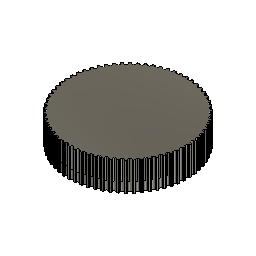
gear_66Z (Autodesk Fusion 360 design; units mm, degrees)
Autodesk Fusion 360 part; units mm, degrees
sketch "Sketch1" plane through (0, 0, 0) normal (0, 0, 1) x (1, 0, 0) in component "gt2 pulley"
  circle A0 centre (0, 0) radius 21.0085 construction
  circle A1 centre (0, 0) radius 20.0045 construction
  line L0 (0, 0) -> (0, 21.0085) construction
  line L1 (0, 0) -> (0.9996, 20.9847) construction
  line L2 (0, 0) -> (1.4058, 20.9614) construction
  circle A2 centre (0, 0) radius 20.7545 construction
  arc A3 (0.3929, 20.6167) -> (0.4663, 20.3219) centre (1.3888, 20.7079) ccw
  circle A4 centre (0, 0) radius 20.6045 construction
  arc A5 (0.2453, 20.753) -> (0, 20.7545) centre (0, 0) ccw
  arc A6 (0.3929, 20.6167) -> (0.2453, 20.753) centre (0.2436, 20.603) ccw
  arc A7 (0.4663, 20.3219) -> (0.9519, 19.9818) centre (0.9783, 20.5362) ccw
  arc A8 (0, 20.7545) -> (-0.2453, 20.753) centre (0, 0) ccw
  arc A9 (-0.2453, 20.753) -> (-0.3929, 20.6167) centre (-0.2436, 20.603) ccw
  arc A10 (-0.4663, 20.3219) -> (-0.3929, 20.6167) centre (-1.3888, 20.7079) ccw
  arc A11 (-0.9519, 19.9818) -> (-0.4663, 20.3219) centre (-0.9783, 20.5362) ccw
  arc A12 (0.9519, 19.9818) -> (-0.9519, 19.9818) centre (0, 0) ccw
  point P0 (1.3888, 20.7079)
  point P1 (0, 20.7545)
  dimension "d18" = 42.0169
  dimension "d19" = 2.727
  dimension "d22" = 1.004
  dimension "d24" = 0.75
  dimension "d26" = 1
  dimension "d27" = 0.15
  dimension "d28" = 0.15
  dimension "d47" = 0.555
  dimension "d52" = 3.812
  constraint coincident A0.centre A1.centre
  constraint coincident A0 L0.end
  constraint vertical L0
  constraint coincident A0 L1.end
  constraint coincident A0 L2.end
  constraint concentric A1 A2
  constraint coincident A1 A7.end
  constraint coincident L1 A7.end
  constraint coincident A2 P0
  constraint coincident L2 P0
  constraint coincident P0 A3.centre
  constraint coincident A2 P1
  constraint coincident L0 P1
  constraint concentric A2 A4
  constraint coincident P1 A5.end
  constraint coincident A4 A6.centre
  constraint coincident A3.start A6.start
  constraint tangent A3 A6
  constraint tangent A3 A7
  constraint symmetric L0 A7.end A11.start
  constraint symmetric L0 A3.start A9.end
  constraint symmetric L0 A3.end A10.start
  constraint symmetric L0 A3 A10
  constraint symmetric L0 A5.start A8.end
  constraint symmetric L0 P1 A5.end
  constraint symmetric L0 A5 A8
  constraint symmetric L0 A6 A9
  constraint symmetric L0 A7 A11
  constraint coincident A1 A11.start
  constraint tangent A1 A7
  constraint coincident L1 A7.centre
  measures "d18" diameter of A0
  measures "d19" angle of L0 L1
  measures "d22" distance of A0 A1
  measures "d24" distance of A1 A2
  measures "d26" radius of A3
  measures "d27" distance of A2 A4
  measures "d28" radius of A6
  measures "d47" radius of A7
extrude "Extrude4" [suppressed] in component "gt2 pulley"
pattern_circular "C-Pattern7" [suppressed] in component "gt2 pulley"
extrude "Extrude3" [suppressed] in component "gt2 pulley"
pattern_circular "C-Pattern6" [suppressed] in component "gt2 pulley"
extrude "Extrude2" [suppressed] in component "gt2 pulley"
pattern_circular "C-Pattern5" [suppressed] in component "gt2 pulley"
extrude "Extrude1" [suppressed] in component "gt2 pulley"
pattern_circular "C-Pattern4" [suppressed] in component "gt2 pulley"
pattern_circular "C-Pattern3" [suppressed] in component "gt2 pulley"
pattern_circular "C-Pattern2" [suppressed] in component "gt2 pulley"
pattern_circular "C-Pattern1" [suppressed] in component "gt2 pulley"
copy_body "Body->Comp1" [suppressed] in component "Component"
copy_body "Body->Comp2" [suppressed] in component "Component'"
copy_body "Body->Comp3" [suppressed] in component "Component''"
copy_body "Body->Comp4" [suppressed] in component "Component'''"
copy_body "Body->Comp5" [suppressed] in component "Component''''"
copy_body "Body->Comp6" [suppressed] in component "Component'''''"
copy_body "Body->Comp7" [suppressed] in component "Component''''''"
copy_body "Body->Comp8" [suppressed] in component "Component'''''''"
copy_body "Body->Comp9" [suppressed] in component "Component''''''''"
copy_body "Body->Comp10" [suppressed] in component "Component'''''''''"
copy_body "Body->Comp11" [suppressed] in component "Component''''''''''"
copy_body "Body->Comp12" [suppressed] in component "Component'''''''''''"
copy_body "Body->Comp13" [suppressed] in component "Component''''''''''''"
copy_body "Body->Comp14" [suppressed] in component "Component'''''''''''''"
copy_body "Body->Comp15" [suppressed] in component "Component''''''''''''''"
copy_body "Body->Comp16" [suppressed] in component "Component'''''''''''''''"
copy_body "Body->Comp17" [suppressed] in component "Component''''''''''''''''"
copy_body "Body->Comp18" [suppressed] in component "Component'''''''''''''''''"
copy_body "Body->Comp19" [suppressed] in component "Component''''''''''''''''''"
copy_body "Body->Comp20" [suppressed] in component "Component'''''''''''''''''''"
extrude "Extrude1'" add sketch "Sketch1" along normal blind 7 makes body 1
pattern_circular "C-Pattern1'" count 66 over 360 about axis through (0, 0, 1.75) along (0, 0, 1) of bodies 1 makes body 2 at (-2.0069, 19.9035, 4.6667) makes body 3 at (-3.8897, 19.6226, 4.6667) makes body 4 at (-5.7374, 19.164, 4.6667) makes body 5 at (-6.7424, 18.834, 2.3333) makes body 6 at (-9.2605, 17.7319, 4.6667) makes body 7 at (-10.1849, 17.2176, 2.3333) makes body 8 at (-11.7754, 16.1715, 2.3333) makes body 9 at (-13.2593, 14.9789, 2.3333) makes body 10 at (-14.6231, 13.6507, 2.3333) makes body 11 at (-15.8545, 12.1989, 2.3333) makes body 12 at (-17.377, 9.9104, 4.6667) makes body 13 at (-18.2404, 8.2138, 4.6667) makes body 14 at (-19.1335, 5.8386, 4.6667) makes body 15 at (-19.4652, 4.6133, 4.6667) makes body 16 at (-19.6819, 3.5779, 2.3333) makes body 17 at (-19.9866, 0.8461, 4.6667) makes body 18 at (-19.9765, -1.0576, 4.6667) makes body 19 at (-19.7855, -2.9517, 4.6667) makes body 20 at (-19.2527, -5.4326, 4.6667) makes body 21 at (-19.1334, -5.8386, 2.3333) makes body 22 at (-17.8766, -8.978, 4.6667) makes body 23 at (-16.9422, -10.6367, 4.6667) makes body 24 at (-16.7135, -10.9926, 2.3333) makes body 25 at (-14.6231, -13.6508, 4.6667) makes body 26 at (-13.7279, -14.5507, 4.6667) makes body 27 at (-11.7754, -16.1715, 4.6667) makes body 28 at (-10.1849, -17.2176, 4.6667) makes body 29 at (-9.0724, -17.8289, 4.6667) makes body 30 at (-6.7424, -18.834, 4.6667) makes body 31 at (-5.5343, -19.2237, 4.6667) makes body 32 at (-4.5103, -19.4894, 2.3333) makes body 33 at (-1.7962, -19.9237, 4.6667) makes body 34 at (0.1058, -20.0042, 4.6667) makes body 35 at (2.6374, -19.8298, 4.6667) makes body 36 at (3.8897, -19.6226, 4.6667) makes body 37 at (6.3425, -18.9724, 4.6667) makes body 38 at (7.5331, -18.5319, 4.6667) makes body 39 at (9.8185, -17.4292, 4.6667) makes body 40 at (10.1849, -17.2176, 2.3333) makes body 41 at (12.449, -15.6589, 4.6667) makes body 42 at (13.2593, -14.9789, 2.3333) makes body 43 at (14.6231, -13.6507, 2.3333) makes body 44 at (15.8545, -12.1989, 2.3333) makes body 45 at (17.6827, -9.3541, 4.6667) makes body 46 at (18.2404, -8.2138, 4.6667) makes body 47 at (19.1335, -5.8386, 4.6667) makes body 48 at (19.2527, -5.4326, 2.3333) makes body 49 at (19.6819, -3.5779, 2.3333) makes body 50 at (19.9329, -1.6908, 2.3333) makes body 51 at (20.0033, 0.2116, 2.3333) makes body 52 at (19.7855, 2.9517, 4.6667) makes body 53 at (19.2527, 5.4326, 4.6667) makes body 54 at (18.8693, 6.6427, 4.6667) makes body 55 at (17.8766, 8.978, 4.6667) makes body 56 at (17.2712, 10.0937, 4.6667) makes body 57 at (16.7135, 10.9926, 2.3333) makes body 58 at (15.5929, 12.5316, 2.3333) makes body 59 at (13.7279, 14.5507, 4.6667) makes body 60 at (11.7754, 16.1715, 4.6667) makes body 61 at (10.1849, 17.2176, 4.6667) makes body 62 at (8.5021, 18.1078, 4.6667) makes body 63 at (6.7424, 18.834, 4.6667) makes body 64 at (6.3425, 18.9724, 2.3333) makes body 65 at (4.5103, 19.4894, 2.3333) makes body 66 at (2.6373, 19.8298, 2.3333)
sketch "Sketch1 (2)" plane through (0, 0, 7) normal (0, 0, 1) x (-1, 0, 0)
  arc A0 (-15.8384, -13.2041) -> (-15.8447, -13.405) centre (-15.7302, -13.308) ccw
  arc A1 (-15.8447, -13.405) -> (-15.5235, -13.7757) centre (0, 0) ccw
  arc A2 (-15.5235, -13.7757) -> (-15.3237, -13.798) centre (-15.4112, -13.6762) ccw
  arc A3 (-15.053, -13.6604) -> (-15.3237, -13.798) centre (-14.7406, -14.6104) ccw
  arc A4 (-14.4779, -13.8047) -> (-15.053, -13.6604) centre (-14.8796, -14.1876) ccw
  arc A5 (-15.7246, -12.3659) -> (-14.4779, -13.8047) centre (0, 0) ccw
  arc A6 (-15.6636, -12.9557) -> (-15.7246, -12.3659) centre (-16.1608, -12.709) ccw
  arc A7 (-15.8384, -13.2041) -> (-15.6636, -12.9557) centre (-16.5595, -12.5113) ccw
  circle A8 centre (0, 0) radius 20.0045
  constraint concentric A1 A8
extrude "Extrude2'" add sketch "Sketch1 (2)" against normal blind 7 contours A5 A8 bodies 1 2 3 4 5 6 7 8 9 10 11 12 13 14 15 16 17 18 19 20 21 22 23 24 25 26 27 28 29 30 31 32 33 34 35 36 37 38 39 40 41 42 43 44 45 46 47 48 49 50 51 52 53 54 55 56 57 58 59 60 61 62 63 64 65 66
extrude "Extrude3'" add 1 faces at (-4.826, 4.6016, 0) along direction (0, 0, -1) blind 3 on bodies 1 bodies 1
component "gear for gt2 v2" placed x (1, 0, 0) y (0, 1, 0) z (0, 0, 1) at (0, 0, 0)
component "gt2 pulley" placed x (1, 0, 0) y (0, 1, 0) z (0, 0, 1) at (0, 0, 0) in component "gear for gt2 v2"
equation "NumTeeth = 66" comment "min 20"
equation "ToothPitch = 2 mm"
equation "PullyDia = NumTeeth * ToothPitch / PI"
equation "ToothAng = ( ( 360 / NumTeeth ) * 1 deg )"
equation "TransOffsetAngle = ToothAng * 0.2"
equation "Sholulder_Radius = 0.15 mm"
equation "Root_Radius = 0.555 mm"
equation "TransRadius = 1 mm"
equation "ToolHeight = 0.75 mm"
equation "PLD = 0.254 mm"
equation "d18 = PullyDia"
equation "d19 = ToothAng / 2"
equation "d22 = PLD + ToolHeight"
equation "d24 = ToolHeight"
equation "d26 = TransRadius"
equation "d27 = Sholulder_Radius"
equation "d31 = NumTeeth"
equation "d33 = NumTeeth"
equation "d35 = NumTeeth"
equation "d37 = NumTeeth"
equation "d41 = NumTeeth"
equation "d45 = NumTeeth"
equation "d47 = Root_Radius"
equation "d50 = NumTeeth"
